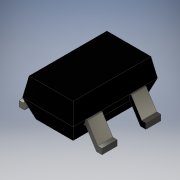
# Autodesk Inventor part: MC_MMM1362
Saved by Autodesk Inventor 2016 (Build 200138000, 138)
## iProperties
Created: 2016-08-30
Part Number: MC_MMM1362
Material: Generic
Document SubType Name: Modeling
Designer: jfixelle
Density: 1 g/cm^3
Appearance: Black
Author: jfixelle
Autodesk Inventor part; units mm, degrees
ref_plane "YZ Plane" through (0, 0, 0) normal (1, 0, 0) x (0, 1, 0)
ref_plane "XZ Plane" through (0, 0, 0) normal (0, 1, 0) x (-1, 0, 0)
ref_plane "XY Plane" through (0, 0, 0) normal (0, 0, 1) x (1, 0, 0)
sketch "Sketch1" plane through (0, 0, 0) normal (0, 1, 0) x (-1, 0, 0)
  line L0 (0.675, 1.125) -> (-0.675, 1.125)
  line L1 (-0.675, 1.125) -> (-0.675, -1.125)
  line L2 (-0.675, -1.125) -> (0.675, -1.125)
  line L3 (0.675, -1.125) -> (0.675, 1.125)
  point P0 (0, 0)
  dimension "d0" = 1.35
  dimension "d1" = 0.675
  dimension "d2" = 2.25
  dimension "d3" = 1.125
  constraints: 8 end point, 2 parallel, 1 horizontal, 1 perpendicular
  measures "d0" distance of L0.start L0.end
  measures "d1" distance from line of L3 point (0, 0)
  measures "d2" distance of L2.end L0.start
  measures "d3" distance from line of L2 point (0, 0)
extrude "Extrusion1" add sketch "Sketch1" along normal blind 1
chamfer "Chamfer1" distance 0.5 angle 10 1 edges at (0.675, 1, 0) measured on face at (0.675, 0.3333, 0.375)
chamfer "Chamfer2" distance 0.5 angle 10 1 edges at (-0.0441, 1, 1.125) measured on face at (-0.225, 0.5, 1.125)
chamfer "Chamfer3" distance 0.5 angle 10 1 edges at (-0.0441, 1, -1.125) measured on face at (-0.225, 0.5, -1.125)
chamfer "Chamfer4" distance 0.5 angle 10 1 edges at (-0.675, 1, 0) measured on face at (-0.675, 0.1667, -0.375)
chamfer "Chamfer5" distance 0.5 angle 20 1 edges at (-0.675, 0, 0) measured on face at (-0.675, 0.3333, 0.375)
chamfer "Chamfer6" distance 0.5 angle 20 1 edges at (0.0907, 0, -1.125) measured on face at (-0.1645, 0.3332, -1.125)
chamfer "Chamfer7" distance 0.5 angle 20 1 edges at (0.675, 0, 0.0907) measured on face at (0.675, 0.3333, -0.3145)
chamfer "Chamfer8" distance 0.5 angle 20 1 edges at (0, 0, 1.125) measured on face at (0.1645, 0.333, 1.125)
sketch "Sketch2" plane through (0, 0, 0) normal (0, 0, 1) x (1, 0, 0)
  line L0 (-0.6745, 0.5) -> (-0.7101, 0.5)
  line L1 (-0.7101, 0.5) -> (-0.993, 0.05)
  line L2 (-0.993, 0.05) -> (-1.1045, 0.05)
  line L3 (-1.1045, 0.05) -> (-1.1045, -0.1)
  line L4 (-1.1045, -0.1) -> (-0.9581, -0.1)
  line L5 (-0.9581, -0.1) -> (-0.6752, 0.35)
  line L6 (-0.6752, 0.35) -> (-0.6745, 0.35)
  line L7 (-0.6745, 0.35) -> (-0.6745, 0.5)
  line L8 (-0.493, 0) -> (0.493, 0) projected
  line L9 (-0.6745, 0.35) -> (-0.5079, 0.35)
  line L10 (-0.5079, 0.35) -> (-0.5079, 0.5)
  line L11 (-0.5079, 0.5) -> (-0.6745, 0.5)
  line L12 (-0.6745, 0.5) -> (-0.6745, 0.35)
  point P0 (0, 0)
  dimension "d30" = 0.15
  dimension "d31" = 0.15
  dimension "d32" = 0.1
  dimension "d33" = 0.43
  dimension "d34" = 0.5
  constraints: 24 end point, 5 parallel, 4 perpendicular, 2 horizontal
  measures "d30" distance of L2.end L3.end
  measures "d31" distance of L6.end L0.start
  measures "d32" distance between parallel lines of L8 L4
  measures "d33" distance between parallel lines of L7 L3
  measures "d34" distance between parallel lines of L8 L0
extrude "Extrusion2" add sketch "Sketch2" along normal mid plane 1.57
mirror "Mirror1" about plane through (0, 0, 0) normal (1, 0, 0) of "Extrusion2"
sketch "Sketch3" plane through (0, 1, 0) normal (0, 1, 0) x (1, 0, 0)
  line L0 (0.675, -0.785) -> (0.675, 0.785) projected
  line L1 (1.3066, 0.385) -> (0.675, 0.385)
  line L2 (0.675, 0.385) -> (0.675, -0.385)
  line L3 (0.675, -0.385) -> (1.3066, -0.385)
  line L4 (1.3066, -0.385) -> (1.3066, 0.385)
  line L5 (-0.675, 0.785) -> (-0.675, -0.785) projected
  line L6 (-0.675, -0.085) -> (-1.3547, -0.085)
  line L7 (-1.3547, -0.085) -> (-1.3547, 0.385)
  line L8 (-1.3547, 0.385) -> (-0.675, 0.385)
  line L9 (-0.675, 0.385) -> (-0.675, -0.085)
  line L10 (-0.993, 0.785) -> (-0.7101, 0.785) projected
  point P0 (0, 0)
  dimension "d38" = 0.77
  dimension "d39" = 0.385
  dimension "d40" = 0.47
  dimension "d41" = 0.4
  constraints: 16 end point, 4 parallel, 2 horizontal, 2 perpendicular, 2 point on line
  measures "d38" distance of L3.end L1.start
  measures "d39" distance from line of point (0, 0) L1
  measures "d40" distance of L6.end L7.end
  measures "d41" distance between parallel lines of L10 L8
extrude "Extrusion3" cut sketch "Sketch3" against normal blind 1.57
body "Solid1"
